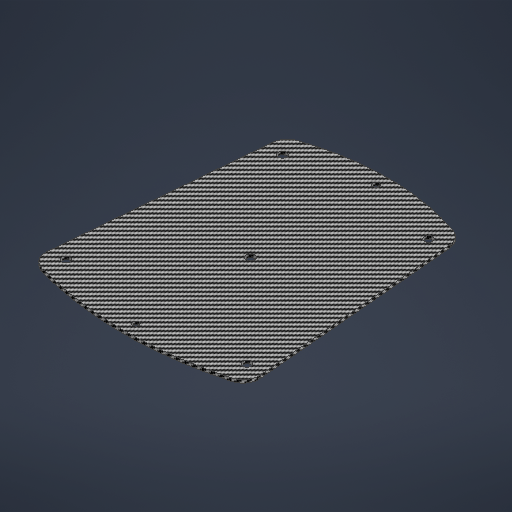
# Autodesk Inventor part: Spiegelhalterung
Saved by Autodesk Inventor 2025.2 (Build 292293000, 293)
## iProperties
Created: 2024-11-26
Part Number: Spiegelhalterung
Material: Generisch
Document SubType Name: Modeling
Designer: Fabian
Density: 1 g/cm^3
Appearance: Kohlenstofffaser
Author: Fabian
Autodesk Inventor part; units mm, degrees
ref_plane "YZ Plane" through (0, 0, 0) normal (1, 0, 0) x (0, 1, 0)
ref_plane "XZ Plane" through (0, 0, 0) normal (0, 1, 0) x (-1, 0, 0)
ref_plane "XY Plane" through (0, 0, 0) normal (0, 0, 1) x (1, 0, 0)
sketch "Skizze1" plane through (0, 0, 0) normal (0, 1, 0) x (-1, 0, 0)
  line L0 (13, 63) -> (-13, 63) construction
  line L1 (0, 63) -> (0, -88) construction
  arc A0 (-35.0888, -80.7018) -> (35.0888, -80.7018) centre (0, 0) ccw construction
  arc A1 (-85.5688, 20.542) -> (-77.3365, -41.9889) centre (0, 0) ccw construction
  arc A2 (77.3365, -41.9889) -> (85.5688, 20.542) centre (0, 0) ccw construction
  line L2 (36.329, -52.1602) -> (44.9364, 46.717) construction
  line L3 (44.9364, 46.717) -> (-44.9364, 46.717) construction
  line L4 (-44.9364, 46.717) -> (-36.329, -52.1602) construction
  line L5 (-36.329, -52.1602) -> (36.329, -52.1602) construction
  line L6 (44.2988, -52.854) -> (52.9063, 46.0232)
  line L7 (44.9364, 54.717) -> (-44.9364, 54.717)
  line L8 (-52.9063, 46.0232) -> (-44.2988, -52.854)
  line L9 (-36.329, -60.1602) -> (36.329, -60.1602)
  arc A3 (36.329, -60.1602) -> (44.2988, -52.854) centre (36.329, -52.1602) ccw
  arc A4 (-44.2988, -52.854) -> (-36.329, -60.1602) centre (-36.329, -52.1602) ccw
  arc A5 (-44.9364, 54.717) -> (-52.9063, 46.0232) centre (-44.9364, 46.717) ccw
  arc A6 (52.9063, 46.0232) -> (44.9364, 54.717) centre (44.9364, 46.717) ccw
  line L10 (43.6628, -60.1602) -> (53.6631, 54.717)
  line L11 (53.6631, 54.717) -> (-53.6631, 54.717)
  line L12 (-53.6631, 54.717) -> (-43.6628, -60.1602)
  line L13 (-43.6628, -60.1602) -> (43.6628, -60.1602)
  arc A7 (-43.6628, -60.1602) -> (43.6628, -60.1602) centre (0, 50.7799) ccw
  arc A8 (53.6631, 54.717) -> (-53.6631, 54.717) centre (0, -114.9743) ccw
  line L14 (0, 63) -> (0, 51)
  line L15 (6, 51) -> (-6, 51)
  line L16 (-6, 51) -> (-6, 63)
  line L17 (-6, 63) -> (6, 63)
  line L18 (6, 63) -> (6, 51)
  line L19 (6, 51) -> (-6, 63) construction
  line L20 (-6, 51) -> (6, 63) construction
  line L21 (0, -68.4432) -> (0, -56.4432)
  line L22 (6, -68.4432) -> (-6, -68.4432)
  line L23 (-6, -68.4432) -> (-6, -56.4432)
  line L24 (-6, -56.4432) -> (6, -56.4432)
  line L25 (6, -56.4432) -> (6, -68.4432)
  line L26 (6, -68.4432) -> (-6, -56.4432) construction
  line L27 (-6, -68.4432) -> (6, -56.4432) construction
  circle A9 centre (0, 0) radius 88
  point P0 (0, 0)
  point P1 (136.7943, -100.6712)
  point P2 (133.0243, -72.1229)
  point P3 (126.2508, -68.622)
  point P4 (131.1382, -105.7457)
  point P5 (170.7312, -118.661)
  point P6 (170.703, -118.661)
  point P7 (165.9867, -123.8079)
  point P8 (170.7158, -118.647)
  point P9 (181.0377, -128.1052)
  point P10 (176.3086, -133.2662)
  point P11 (-44.9364, 54.717)
  point P12 (-44.9364, 54.717)
  point P13 (0, 57)
  point P14 (0, -62.4432)
  point P15 (0, -62.4432)
  point P16 (0, 57)
  point P17 (6, -68.2921)
  point P18 (-6, -68.2921)
  point P19 (-6, 62.8988)
  point P20 (6, 62.8988)
  dimension "d27" = 72.6579
  dimension "d28" = 89.8728
  dimension "d29" = 8
  dimension "d30" = 8
  dimension "d38" = 8
  dimension "d43" = 12
  dimension "d44" = 12
  dimension "d45" = 12
  dimension "d46" = 12
  constraints: 56 end point, 21 point on circle, 10 centre point, 8 tangent, 7 midpoint, 7 parallel, 4 coincident, 4 equal radius, 4 symmetric about line, 3 horizontal, 3 point on line, 2 perpendicular, 1 vertical, 7 other
  measures "d27" distance of L4.end L2.start
  measures "d28" distance of L2.end L3.end
  measures "d29" distance between parallel lines of L5 L9
  measures "d30" radius of A3
  measures "d38" distance between parallel lines of L5 L13
  measures "d43" distance of L1.start L14.end
  measures "d44" distance of L16.end L17.end
  measures "d45" distance of L21.start L21.end
  measures "d46" distance of L23.end L24.end
extrude "Extrusion1" add sketch "Skizze1" against normal blind 1.5 contours A3 L9 L25 L24 L23 A4 L8 A5 L7 L16 L15 L18 A6 L6 | L10 L13 A3 | A6 L11 L10 | L13 A7 L25 L9 | L7 L18 A8 L11 | L25 A7 L21 L9 | L9 L21 L24 L25 | L18 L15 L14 L7 | L7 L14 A8 L18 | L21 A7 L23 L9 | L9 L23 L24 L21 | L14 L15 L16 L7 | L7 L16 A8 L14 | L23 A7 L13 L9 | L7 L11 A8 L16 | L13 L12 A4 | A5 L12 L11
hole "Bohrung1" at (36.329, 0, -52.1602) at (44.9364, 0, 46.717) at (0, 0, 0) at (-36.329, 0, -52.1602) at (-44.9364, 0, 46.717) direction (0, -1, 0) diameter 4.2 depth 1.5
hole "Bohrung2" at (0, 0, 57) at (0, 0, -62.4432) direction (0, -1, 0) diameter 3.2 depth 1.5
fillet "Rundung2" radius 8 4 edges at (53.6631, -0.75, 54.717) (43.6628, -0.75, -60.1602) (-43.6628, -0.75, -60.1602) (-53.6631, -0.75, 54.717)
